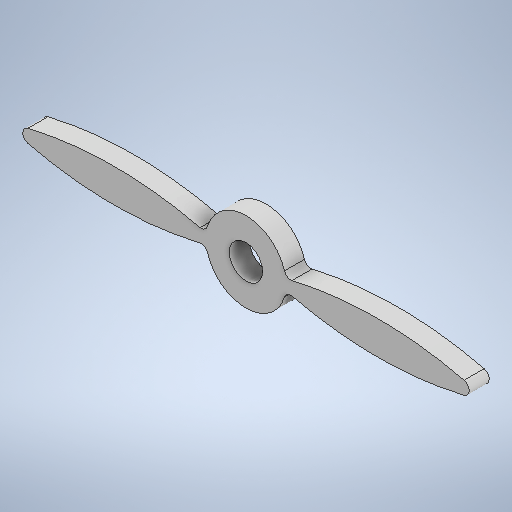
# Autodesk Inventor part: HELICE
Saved by Autodesk Inventor 2025.1 (Build 291241000, 241)
## iProperties
Created: 2024-10-18
Part Number: HELICE
Material: Genérico
Document SubType Name: Modeling
Designer: Aluno
Density: 1 g/cm^3
Appearance: Padrão
Author: Aluno
Autodesk Inventor part; units mm, degrees
ref_plane "YZ Plane" through (0, 0, 0) normal (1, 0, 0) x (0, 1, 0)
ref_plane "XZ Plane" through (0, 0, 0) normal (0, 1, 0) x (-1, 0, 0)
ref_plane "XY Plane" through (0, 0, 0) normal (0, 0, 1) x (1, 0, 0)
sketch "Esboço1" plane through (0, 0, 0) normal (0, 0, 1) x (1, 0, 0)
  arc A0 (-32.6171, 0.9719) -> (-32.6171, -0.9719) centre (-32.3816, 0) ccw
  line L0 (-6, 0) -> (-7, 0)
  arc A1 (-6.8571, 0.9897) -> (-5.7551, 1.6967) centre (-6.7143, 1.9795) ccw
  arc A2 (-5.7551, -1.6967) -> (-7.0345, -1.0321) centre (-6.7143, -1.9795) ccw
  arc A3 (-6.8571, 0.9897) -> (-32.6171, 0.9719) centre (-19.7001, -52.3443) ccw
  arc A4 (-32.6171, -0.9719) -> (-7.0345, -1.0321) centre (-19.7001, 52.3443) ccw
  arc A5 (0, 2.5) -> (0, -2.5) centre (0, 0) ccw
  arc A6 (32.6171, -0.9719) -> (32.6171, 0.9719) centre (32.3816, 0) ccw
  line L1 (6, 0) -> (7, 0)
  arc A7 (5.7551, 1.6967) -> (6.8571, 0.9897) centre (6.7143, 1.9795) ccw
  arc A8 (7.0345, -1.0321) -> (5.7551, -1.6967) centre (6.7143, -1.9795) ccw
  arc A9 (32.6171, 0.9719) -> (6.8571, 0.9897) centre (19.7001, -52.3443) ccw
  arc A10 (7.0345, -1.0321) -> (32.6171, -0.9719) centre (19.7001, 52.3443) ccw
  arc A11 (0, -2.5) -> (0, 2.5) centre (0, 0) ccw
  arc A12 (0, 6) -> (-5.7551, 1.6967) centre (0, 0) ccw
  arc A13 (-5.7551, -1.6967) -> (0, -6) centre (0, 0) ccw
  arc A14 (0, -6) -> (5.7551, -1.6967) centre (0, 0) ccw
  arc A15 (5.7551, 1.6967) -> (0, 6) centre (0, 0) ccw
  point P0 (-6.7143, 2.9795)
  point P1 (-6.7143, 0.9795)
  point P2 (-6.7143, -0.9795)
  point P3 (-6.7143, -2.9795)
  point P4 (6.7143, 2.9795)
  point P5 (6.7143, 0.9795)
  point P6 (6.7143, -0.9795)
  point P7 (6.7143, -2.9795)
  constraints: 40 point on circle, 16 centre point, 4 end point, 2 coincident, 2 tangent
extrude "Extrusão1" add sketch "Esboço1" along normal blind 3
